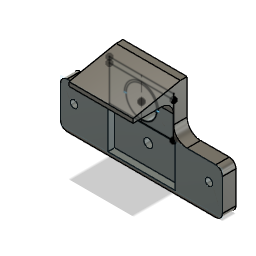
Camera and Ultrasonic Sensor mount v3 (Autodesk Fusion 360 design; units mm, degrees)
Autodesk Fusion 360 part; units mm, degrees
sketch "Sketch1" plane through (0, 0, 0) normal (0, 0, 1) x (1, 0, 0)
  line L0 (0, 0) -> (120, 0)
  line L1 (120, 0) -> (120, 32)
  line L2 (120, 32) -> (0, 32)
  line L3 (0, 32) -> (0, 0)
  dimension "d1" = 120
  dimension "d2" = 32
  constraint horizontal L0
  constraint vertical L1
  constraint horizontal L2
  constraint vertical L3
  constraint coincident L0.start L3.end
  measures "d1" distance of L1.end L2.end
  measures "d2" distance of L0.start L2.end
extrude "Extrude1" add sketch "Sketch1" along normal blind 10
sketch "Sketch2" plane through (0, 0, 10) normal (0, 0, 1) x (1, 0, 0)
  line L0 (0, 32) -> (0, 0)
  line L1 (0, 0) -> (120, 0)
  line L2 (120, 0) -> (120, 32)
  line L3 (120, 32) -> (0, 32)
  line L4 (60, 32) -> (60, 0) construction
  circle A0 centre (10, 18.5) radius 2.75
  circle A1 centre (110, 18.5) radius 2.75
  dimension "d5" = 100
  dimension "d6" = 13.5
  dimension "d7" = 5.5
  dimension "d8" = 5.5
  dimension "d9" = 50
  constraint midpoint L3 L4.start
  constraint midpoint L1 L4.end
  measures "d5" distance of A0.centre A1.centre
  measures "d6" distance of L3 A0.centre
  measures "d7" diameter of A0
  measures "d8" diameter of A1
  measures "d9" distance of L4 A0.centre
extrude "Extrude2" cut sketch "Sketch2" against normal blind 10 contours A0 | A1
sketch "Sketch3" plane through (0, 0, 10) normal (0, 0, 1) x (1, 0, 0)
  circle A0 centre (10, 18.5) radius 2.75
  circle A1 centre (110, 18.5) radius 2.75
  line L0 (0, 32) -> (0, 0)
  line L1 (0, 0) -> (120, 0)
  line L2 (120, 0) -> (120, 32)
  line L3 (120, 32) -> (0, 32)
  line L4 (60, 32) -> (60, 0) construction
  line L5 (35.125, 31.5) -> (84.875, 31.5)
  line L6 (84.875, 31.5) -> (84.875, 0.5)
  line L7 (84.875, 0.5) -> (35.125, 0.5)
  line L8 (35.125, 0.5) -> (35.125, 31.5)
  line L9 (0, 16) -> (120, 16) construction
  line L10 (84.875, 0.5) -> (35.125, 31.5) construction
  circle A2 centre (60, 16) radius 3.25
  point P0 (60, 16)
  dimension "d12" = 49.75
  dimension "d13" = 31
  dimension "d16" = 6.5
  constraint midpoint L3 L4.start
  constraint midpoint L1 L4.end
  constraint horizontal L5
  constraint vertical L6
  constraint horizontal L7
  constraint vertical L8
  constraint midpoint L0 L9.start
  constraint midpoint L2 L9.end
  constraint midpoint L4 P0
  constraint midpoint L10 P0
  constraint coincident P0 A2.centre
  measures "d12" distance of L5.start L5.end
  measures "d13" distance of L5.start L7.end
  measures "d16" diameter of A2
extrude "Extrude3" cut sketch "Sketch3" against normal blind 5 contours L5 L6 L7 L8 | A2
extrude "Extrude4" cut sketch "Sketch3" against normal blind 10 contours A2
sketch "Sketch5" plane through (0, 32, 0) normal (0, 1, 0) x (-1, 0, 0)
  line L0 (-120, 0) -> (0, 0)
  line L1 (0, 0) -> (0, 10)
  line L2 (0, 10) -> (-120, 10)
  line L3 (-120, 10) -> (-120, 0)
  line L4 (-60, 0) -> (-60, 10)
  line L5 (-36.25, 0) -> (-83.75, 0)
  line L6 (-83.75, 0) -> (-83.75, 10)
  line L7 (-83.75, 10) -> (-36.25, 10)
  line L8 (-36.25, 10) -> (-36.25, 0)
  dimension "d19" = 47.5
  constraint midpoint L0 L4.start
  constraint midpoint L2 L4.end
  constraint horizontal L5
  constraint vertical L6
  constraint horizontal L7
  constraint vertical L8
  constraint coincident L2 L6.end
  constraint coincident L0 L5.start
  constraint midpoint L4.start L5
  measures "d19" distance of L5.start L5.end
extrude "Extrude5" add sketch "Sketch5" along normal blind 30 contours L0 L2 L4 L5 L6 L7 | L0 L2 L4 L5 L7 L8
sketch "Sketch6" plane through (0, 0, 10) normal (0, 0, 1) x (1, 0, 0)
  line L0 (84.875, 31.5) -> (84.875, 0.5)
  line L1 (84.875, 0.5) -> (35.125, 0.5)
  line L2 (35.125, 0.5) -> (35.125, 31.5)
  line L3 (35.125, 31.5) -> (84.875, 31.5)
  circle A0 centre (10, 18.5) radius 2.75
  circle A1 centre (110, 18.5) radius 2.75
  line L4 (0, 32) -> (0, 0)
  line L5 (0, 0) -> (120, 0)
  line L6 (120, 0) -> (120, 32)
  line L7 (120, 32) -> (83.75, 32)
  line L8 (83.75, 32) -> (83.75, 62)
  line L9 (83.75, 62) -> (36.25, 62)
  line L10 (36.25, 62) -> (36.25, 32)
  line L11 (36.25, 32) -> (0, 32)
  line L12 (36.25, 62) -> (83.75, 62)
  line L13 (83.75, 62) -> (83.75, 32)
  line L14 (83.75, 32) -> (36.25, 32)
  line L15 (36.25, 32) -> (36.25, 62)
  line L16 (60, 32) -> (60, 62) construction
  circle A2 centre (60, 45) radius 11.4
  line L17 (36.25, 58) -> (83.75, 58)
  line L18 (47.375, 45) -> (48.6, 45)
  line L19 (72.625, 45) -> (71.4, 45)
  arc A3 (72.625, 45) -> (47.375, 45) centre (60, 45) ccw
  dimension "d22" = 22.8
  dimension "d23" = 13
  dimension "d24" = 13
  dimension "d40" = 25.25
  constraint horizontal L12
  constraint vertical L13
  constraint horizontal L14
  constraint vertical L15
  constraint coincident L7.end L8.start
  constraint coincident L9.end L10.start
  constraint midpoint L14 L16.start
  constraint midpoint L9 L16.end
  constraint coincident L16 A2.centre
  constraint coincident L10 L17.start
  constraint coincident L8 L17.end
  constraint perpendicular L8 L17
  constraint concentric A2 A3
  constraint coincident A2 L18.end
  constraint perpendicular L16 L18
  constraint coincident A2 L19.end
  constraint parallel L18 L19
  measures "d22" diameter of A2
  measures "d23" distance of L14 A2.centre
  measures "d24" distance of A2.centre L17
  measures "d40" diameter of A3
extrude "Extrude6" cut sketch "Sketch6" against normal blind 10 contours A2
extrude "Extrude7" add 1 faces at (67.9167, 62, 6.6667) along direction (0, 1, 0) blind 6
fillet "Fillet1" radius 10 1 edges at (83.75, 32, 5)
fillet "Fillet1" radius 10 1 edges at (36.25, 32, 5)
sketch "Sketch7" plane through (0, 0, 10) normal (0, 0, 1) x (1, 0, 0)
  circle A0 centre (60, 45) radius 11.4
  line L0 (84.875, 31.5) -> (84.875, 0.5)
  line L1 (84.875, 0.5) -> (35.125, 0.5)
  line L2 (35.125, 0.5) -> (35.125, 31.5)
  line L3 (35.125, 31.5) -> (84.875, 31.5)
  circle A1 centre (10, 18.5) radius 2.75
  circle A2 centre (110, 18.5) radius 2.75
  line L4 (0, 32) -> (0, 0)
  line L5 (0, 0) -> (120, 0)
  line L6 (120, 0) -> (120, 32)
  line L7 (120, 32) -> (93.75, 32)
  arc A3 (83.75, 42) -> (93.75, 32) centre (93.75, 42) ccw
  line L8 (83.75, 42) -> (83.75, 68)
  line L9 (83.75, 68) -> (36.25, 68)
  line L10 (36.25, 68) -> (36.25, 42)
  arc A4 (26.25, 32) -> (36.25, 42) centre (26.25, 42) ccw
  line L11 (26.25, 32) -> (0, 32)
  line L12 (36.25, 68) -> (83.75, 68)
  line L13 (83.75, 68) -> (83.75, 58)
  line L14 (83.75, 58) -> (36.25, 58)
  line L15 (36.25, 58) -> (36.25, 68)
  dimension "d33" = 10
  constraint horizontal L12
  constraint vertical L13
  constraint horizontal L14
  constraint vertical L15
  constraint coincident L8 L13.end
  constraint coincident L9.end L10.start
  measures "d33" distance of L9.end L14.end
extrude "Extrude8" add sketch "Sketch7" along normal blind 30 contours L8 L9 L10 L12 L13 L14 L15
chamfer "Chamfer1" distance 7 distance2 35 1 edges at (60, 68, 40) measured on face at (67.9167, 61.3333, 40)
fillet "Fillet2" radius 9 1 edges at (60, 58, 10)
extrude "Extrude9" cut sketch "Sketch6" along normal blind 13 contours A2 L18 L19 A3
fillet "Fillet3" radius 5 4 edges at (120, 32, 5) (120, 0, 5) (0, 32, 5) (0, 0, 5)
move_face "OffsetFaces1" offset 1.75 1 faces at (41.6667, 0, 3.3333)
